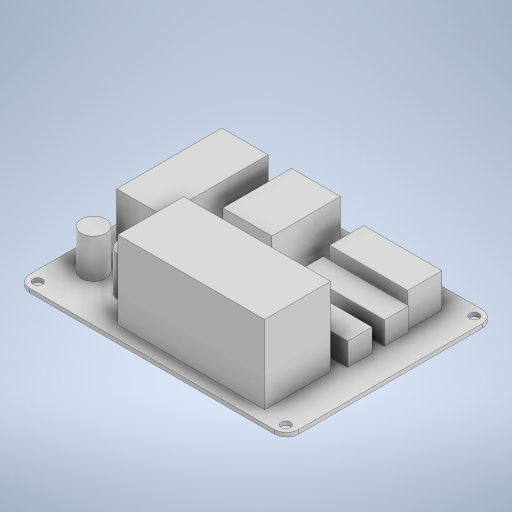
# Autodesk Inventor part: 3waysplitter
Saved by Autodesk Inventor 2023 (Build 270158000, 158)
## iProperties
Created: 2022-07-14
Part Number: 3waysplitter
Material: Generic
Document SubType Name: Modeling
Designer: Fuzzyfish
Density: 1 g/cm^3
Appearance: Default
Author: Fuzzyfish
Autodesk Inventor part; units mm, degrees
ref_plane "YZ Plane" through (0, 0, 0) normal (1, 0, 0) x (0, 1, 0)
ref_plane "XZ Plane" through (0, 0, 0) normal (0, 1, 0) x (-1, 0, 0)
ref_plane "XY Plane" through (0, 0, 0) normal (0, 0, 1) x (1, 0, 0)
sketch "Sketch1" plane through (0, 0, 0) normal (0, 1, 0) x (-1, 0, 0)
  line L0 (0, 0) -> (110, 0)
  line L1 (110, 0) -> (110, -85)
  line L2 (110, -85) -> (0, -85)
  line L3 (0, -85) -> (0, 0)
  dimension "d0" = 85
  dimension "d1" = 110
  constraints: 8 end point, 2 parallel, 1 horizontal, 1 perpendicular
  measures "d0" distance of L0.end L1.end
  measures "d1" distance of L1.end L2.end
extrude "Extrusion1" add sketch "Sketch1" along normal blind 1.6
fillet "Fillet1" radius 5 4 edges at (0, 0.8, -85) (0, 0.8, 0) (-110, 0.8, 0) (-110, 0.8, -85)
sketch "Sketch2" plane through (0, 1.6, 0) normal (0, 1, 0) x (1, 0, 0)
  circle A0 centre (-4.3, 4) radius 1.95
  circle A1 centre (-4.3, 81) radius 1.95
  circle A2 centre (-105.7, 81) radius 1.95
  circle A3 centre (-105.7, 4) radius 1.95
  line L0 (-110, 80) -> (-110, 5) projected
  line L1 (-5, 85) -> (-105, 85) projected
  line L2 (-105, 0) -> (-5, 0) projected
  line L3 (0, 5) -> (0, 80) projected
  point P0 (0, 0)
  dimension "d5" = 3.9
  dimension "d6" = 3.9
  dimension "d7" = 3.9
  dimension "d8" = 3.9
  dimension "d9" = 4.3
  dimension "d10" = 4
  dimension "d11" = 4.3
  dimension "d12" = 4
  dimension "d13" = 4.3
  dimension "d14" = 4
  dimension "d15" = 4.3
  dimension "d16" = 4
  constraints: 4 centre point
  measures "d5" diameter of A3
  measures "d6" diameter of A2
  measures "d7" diameter of A0
  measures "d8" diameter of A1
  measures "d9" distance from line of L0 A2.centre
  measures "d10" distance from line of L1 A2.centre
  measures "d11" distance from line of L0 A3.centre
  measures "d12" distance from line of L2 A3.centre
  measures "d13" distance from line of L3 A0.centre
  measures "d14" distance from line of L2 A0.centre
  measures "d15" distance from line of L3 A1.centre
  measures "d16" distance from line of L1 A1.centre
extrude "Extrusion2" cut sketch "Sketch2" against normal through all
sketch "Sketch3" plane through (0, 1.6, 0) normal (0, 1, 0) x (1, 0, 0)
  circle A0 centre (-82.85, 19.05) radius 5.05
  circle A1 centre (-97.95, 19.05) radius 5.05
  line L0 (-105, 0) -> (-5, 0) projected
  line L1 (-110, 80) -> (-110, 5) projected
  point P0 (0, 0)
  dimension "d19" = 10.1
  dimension "d20" = 10.1
  dimension "d21" = 19.05
  dimension "d22" = 19.05
  dimension "d23" = 12.05
  dimension "d24" = 15.1
  constraints: 2 centre point
  measures "d19" diameter of A0
  measures "d20" diameter of A1
  measures "d21" distance from line of L0 A1.centre
  measures "d22" distance from line of L0 A0.centre
  measures "d23" distance from line of L1 A1.centre
  measures "d24" distance of A0.centre A1.centre
extrude "Extrusion3" add sketch "Sketch3" along normal blind 16
sketch "Sketch4" plane through (0, 1.6, 0) normal (0, 1, 0) x (1, 0, 0)
  line L0 (-14, 5) -> (-74, 5)
  line L1 (-74, 5) -> (-74, 32)
  line L2 (-74, 32) -> (-14, 32)
  line L3 (-14, 32) -> (-14, 5)
  line L4 (-105, 0) -> (-5, 0) projected
  line L5 (0, 5) -> (0, 80) projected
  point P0 (0, 0)
  dimension "d27" = 60
  dimension "d28" = 27
  dimension "d29" = 5
  dimension "d30" = 14
  constraints: 8 end point, 2 parallel, 1 horizontal, 1 perpendicular
  measures "d27" distance of L0.start L0.end
  measures "d28" distance of L2.end L0.start
  measures "d29" distance between parallel lines of L4 L0
  measures "d30" distance between parallel lines of L5 L3
extrude "Extrusion4" add sketch "Sketch4" along normal blind 32
sketch "Sketch5" plane through (0, 1.6, 0) normal (0, 1, 0) x (1, 0, 0)
  line L0 (-81.5, 31) -> (-100.5, 31)
  line L1 (-100.5, 31) -> (-100.5, 74)
  line L2 (-100.5, 74) -> (-81.5, 74)
  line L3 (-81.5, 74) -> (-81.5, 31)
  line L4 (-110, 80) -> (-110, 5) projected
  line L5 (-5, 85) -> (-105, 85) projected
  point P0 (0, 0)
  dimension "d33" = 9.5
  dimension "d34" = 19
  dimension "d35" = 43
  dimension "d36" = 11
  constraints: 8 end point, 2 parallel, 1 horizontal, 1 perpendicular
  measures "d33" distance between parallel lines of L4 L1
  measures "d34" distance of L0.start L0.end
  measures "d35" distance of L0.end L1.end
  measures "d36" distance between parallel lines of L5 L2
extrude "Extrusion5" add sketch "Sketch5" along normal blind 22
sketch "Sketch6" plane through (0, 1.6, 0) normal (0, 1, 0) x (1, 0, 0)
  line L0 (-49.5, 34) -> (-75.5, 34)
  line L1 (-75.5, 34) -> (-75.5, 46)
  line L2 (-75.5, 46) -> (-49.5, 46)
  line L3 (-49.5, 46) -> (-49.5, 34)
  line L4 (-74, 48) -> (-54, 48)
  line L5 (-54, 48) -> (-54, 76)
  line L6 (-54, 76) -> (-74, 76)
  line L7 (-74, 76) -> (-74, 48)
  line L8 (-13, 62.5) -> (-45, 62.5)
  line L9 (-45, 62.5) -> (-45, 76.5)
  line L10 (-45, 76.5) -> (-13, 76.5)
  line L11 (-13, 76.5) -> (-13, 62.5)
  line L12 (-12, 52) -> (-47, 52)
  line L13 (-47, 52) -> (-47, 62)
  line L14 (-47, 62) -> (-12, 62)
  line L15 (-12, 62) -> (-12, 52)
  line L16 (-12, 37) -> (-47, 37)
  line L17 (-47, 37) -> (-47, 47)
  line L18 (-47, 47) -> (-12, 47)
  line L19 (-12, 47) -> (-12, 37)
  line L20 (-5, 85) -> (-105, 85) projected
  line L21 (-81.5, 31) -> (-81.5, 74) projected
  line L22 (-14, 32) -> (-74, 32) projected
  line L23 (0, 5) -> (0, 80) projected
  point P0 (0, 0)
  dimension "d39" = 20
  dimension "d40" = 28
  dimension "d41" = 9
  dimension "d42" = 2
  dimension "d43" = 12
  dimension "d44" = 26
  dimension "d45" = 6
  dimension "d46" = 7.5
  dimension "d47" = 35
  dimension "d48" = 35
  dimension "d49" = 10
  dimension "d50" = 10
  dimension "d51" = 5
  dimension "d52" = 12
  dimension "d53" = 12
  dimension "d54" = 5
  dimension "d55" = 32
  dimension "d56" = 14
  dimension "d57" = 8.5
  dimension "d58" = 13
  constraints: 40 end point, 10 parallel, 5 horizontal, 5 perpendicular
  measures "d39" distance of L5.end L6.end
  measures "d40" distance of L4.end L5.end
  measures "d41" distance between parallel lines of L20 L6
  measures "d42" distance between parallel lines of L2 L4
  measures "d43" distance between parallel lines of L2 L0
  measures "d44" distance of L0.start L0.end
  measures "d45" distance between parallel lines of L21 L1
  measures "d46" distance between parallel lines of L21 L7
  measures "d47" distance of L17.end L18.end
  measures "d48" distance of L12.start L12.end
  measures "d49" distance of L14.end L12.start
  measures "d50" distance of L18.end L16.start
  measures "d51" distance between parallel lines of L22 L16
  measures "d52" distance between parallel lines of L23 L19
  measures "d53" distance between parallel lines of L23 L15
  measures "d54" distance between parallel lines of L18 L12
  measures "d55" distance of L8.start L8.end
  measures "d56" distance of L10.end L8.start
  measures "d57" distance between parallel lines of L20 L10
  measures "d58" distance between parallel lines of L23 L11
extrude "Extrusion6" add sketch "Sketch6" along normal blind 20 contours L7 L6 L5 L4
extrude "Extrusion7" add sketch "Sketch6" along normal blind 12 contours L0 L1 L2 L3
extrude "Extrusion8" add sketch "Sketch6" along normal blind 9.3 contours L12 L13 L14 L15 | L16 L17 L18 L19
extrude "Extrusion9" add sketch "Sketch6" along normal blind 14 contours L8 L9 L10 L11
equation "\"d6\" = d5"
equation "\"d7\" = d5"
equation "\"d8\" = d7"
equation "\"d11\" = d9"
equation "\"d12\" = d10"
equation "\"d13\" = d9"
equation "\"d14\" = d12"
equation "\"d15\" = d13"
equation "\"d16\" = d14"
equation "\"d19\" = d20"
equation "\"d22\" = d21"
equation "\"d48\" = d47"
equation "\"d50\" = d49"
equation "\"d53\" = d52"
body "Solid1"
